Autodesk Fusion 360 part; units mm, degrees
(part 2 of 2)
  arc A35 (2.9933, 35.5014) -> (4.0928, 36.0294) centre (3.2566, 36.3621) ccw
  arc A36 (2.9933, 35.5014) -> (2.3013, 35.6868) centre (0, 25.7143) ccw
  arc A37 (1.6131, 36.6939) -> (2.3013, 35.6868) centre (2.5036, 36.5638) ccw
  line L18 (1.6131, 36.6939) -> (1.7553, 37.6675)
  spline S18 degree 5 poles (1.7553, 37.6675) (1.7565, 37.6761) (1.7588, 37.6933) (1.7613, 37.7191) (1.7631, 37.7537) (1.7633, 37.797) (1.7619, 37.8405) (1.7595, 37.8841) (1.7567, 37.9278) (1.7535, 37.9715) (1.7499, 38.0152) (1.7458, 38.059) (1.741, 38.1028) (1.7355, 38.1467) (1.7292, 38.1906) (1.7222, 38.2345) (1.7147, 38.2784) (1.7066, 38.3224) (1.698, 38.3663) (1.6891, 38.4103) (1.6797, 38.4543) (1.6698, 38.4982) (1.6595, 38.5422) (1.6487, 38.5862) (1.6374, 38.6301) (1.6257, 38.6741) (1.6135, 38.7181) (1.6009, 38.762) (1.5879, 38.8059) (1.5745, 38.8498) (1.5607, 38.8937) (1.5466, 38.9376) (1.532, 38.9814) (1.517, 39.0253) (1.5016, 39.0691) (1.4859, 39.1128) (1.4697, 39.1566) (1.4532, 39.2003) (1.4364, 39.244) (1.4192, 39.2876) (1.4016, 39.3312) (1.3836, 39.3748) (1.3654, 39.4183) (1.3467, 39.4618) (1.3277, 39.5053) (1.3084, 39.5487) (1.2887, 39.592) (1.2687, 39.6354) (1.2483, 39.6786) (1.2277, 39.7219) (1.2066, 39.765) (1.1853, 39.8081) (1.1636, 39.8512) (1.1416, 39.8942) (1.1193, 39.9372) (1.0967, 39.9801) (1.0738, 40.0229) (1.0505, 40.0657) (1.0269, 40.1084) (1.003, 40.151) (0.9788, 40.1936) (0.9543, 40.2361) (0.9295, 40.2786) (0.9044, 40.321) (0.879, 40.3633) (0.8533, 40.4055) (0.8273, 40.4477) (0.801, 40.4898) (0.7744, 40.5318) (0.7475, 40.5738) (0.7203, 40.6156) (0.6983, 40.6491) (0.6817, 40.6741) (0.6706, 40.6908) (0.665, 40.6991) knots 0 0 0 0 0 0 0.01428571 0.02857143 0.04285714 0.05714286 0.07142857 0.08571429 0.1 0.11428571 0.12857143 0.14285714 0.15714286 0.17142857 0.18571429 0.2 0.21428571 0.22857143 0.24285714 0.25714286 0.27142857 0.28571429 0.3 0.31428571 0.32857143 0.34285714 0.35714286 0.37142857 0.38571429 0.4 0.41428571 0.42857143 0.44285714 0.45714286 0.47142857 0.48571429 0.5 0.51428571 0.52857143 0.54285714 0.55714286 0.57142857 0.58571429 0.6 0.61428571 0.62857143 0.64285714 0.65714286 0.67142857 0.68571429 0.7 0.71428571 0.72857143 0.74285714 0.75714286 0.77142857 0.78571429 0.8 0.81428571 0.82857143 0.84285714 0.85714286 0.87142857 0.88571429 0.9 0.91428571 0.92857143 0.94285714 0.95714286 0.97142857 0.98571429 1 1 1 1 1 1
  arc A38 (0.665, 40.6991) -> (-0.665, 40.6991) centre (0, 25.7143) ccw
  spline S19 degree 5 poles (-0.665, 40.6991) (-0.6706, 40.6908) (-0.6817, 40.6741) (-0.6983, 40.6491) (-0.7203, 40.6156) (-0.7475, 40.5738) (-0.7744, 40.5318) (-0.801, 40.4898) (-0.8273, 40.4477) (-0.8533, 40.4055) (-0.879, 40.3633) (-0.9044, 40.321) (-0.9295, 40.2786) (-0.9543, 40.2361) (-0.9788, 40.1936) (-1.003, 40.151) (-1.0269, 40.1084) (-1.0505, 40.0657) (-1.0738, 40.0229) (-1.0967, 39.9801) (-1.1193, 39.9372) (-1.1416, 39.8942) (-1.1636, 39.8512) (-1.1853, 39.8081) (-1.2066, 39.765) (-1.2277, 39.7219) (-1.2483, 39.6786) (-1.2687, 39.6354) (-1.2887, 39.592) (-1.3084, 39.5487) (-1.3277, 39.5053) (-1.3467, 39.4618) (-1.3654, 39.4183) (-1.3836, 39.3748) (-1.4016, 39.3312) (-1.4192, 39.2876) (-1.4364, 39.244) (-1.4532, 39.2003) (-1.4697, 39.1566) (-1.4859, 39.1128) (-1.5016, 39.0691) (-1.517, 39.0253) (-1.532, 38.9814) (-1.5466, 38.9376) (-1.5607, 38.8937) (-1.5745, 38.8498) (-1.5879, 38.8059) (-1.6009, 38.762) (-1.6135, 38.7181) (-1.6257, 38.6741) (-1.6374, 38.6301) (-1.6487, 38.5862) (-1.6595, 38.5422) (-1.6698, 38.4982) (-1.6797, 38.4543) (-1.6891, 38.4103) (-1.698, 38.3663) (-1.7066, 38.3224) (-1.7147, 38.2784) (-1.7222, 38.2345) (-1.7292, 38.1906) (-1.7355, 38.1467) (-1.741, 38.1028) (-1.7458, 38.059) (-1.7499, 38.0152) (-1.7535, 37.9715) (-1.7567, 37.9278) (-1.7595, 37.8841) (-1.7619, 37.8405) (-1.7633, 37.797) (-1.7631, 37.7537) (-1.7613, 37.7191) (-1.7588, 37.6933) (-1.7565, 37.6761) (-1.7553, 37.6675) knots -1 -1 -1 -1 -1 -1 -0.98571429 -0.97142857 -0.95714286 -0.94285714 -0.92857143 -0.91428571 -0.9 -0.88571429 -0.87142857 -0.85714286 -0.84285714 -0.82857143 -0.81428571 -0.8 -0.78571429 -0.77142857 -0.75714286 -0.74285714 -0.72857143 -0.71428571 -0.7 -0.68571429 -0.67142857 -0.65714286 -0.64285714 -0.62857143 -0.61428571 -0.6 -0.58571429 -0.57142857 -0.55714286 -0.54285714 -0.52857143 -0.51428571 -0.5 -0.48571429 -0.47142857 -0.45714286 -0.44285714 -0.42857143 -0.41428571 -0.4 -0.38571429 -0.37142857 -0.35714286 -0.34285714 -0.32857143 -0.31428571 -0.3 -0.28571429 -0.27142857 -0.25714286 -0.24285714 -0.22857143 -0.21428571 -0.2 -0.18571429 -0.17142857 -0.15714286 -0.14285714 -0.12857143 -0.11428571 -0.1 -0.08571429 -0.07142857 -0.05714286 -0.04285714 -0.02857143 -0.01428571 0 0 0 0 0 0
  line L19 (-1.7553, 37.6675) -> (-1.6131, 36.6939)
  arc A39 (-2.3013, 35.6868) -> (-1.6131, 36.6939) centre (-2.5036, 36.5638) ccw
  arc A40 (-2.3013, 35.6868) -> (-2.9933, 35.5014) centre (0, 25.7143) ccw
  arc A41 (-4.0928, 36.0294) -> (-2.9933, 35.5014) centre (-3.2566, 36.3621) ccw
  line L20 (-4.0928, 36.0294) -> (-4.4565, 36.9437)
  spline S20 degree 5 poles (-4.4565, 36.9437) (-4.4597, 36.9518) (-4.4664, 36.9678) (-4.4771, 36.9914) (-4.4928, 37.0223) (-4.5143, 37.0599) (-4.5373, 37.0969) (-4.5611, 37.1335) (-4.5854, 37.1698) (-4.6101, 37.2061) (-4.635, 37.2422) (-4.6605, 37.278) (-4.6865, 37.3136) (-4.7132, 37.3488) (-4.7406, 37.3837) (-4.7686, 37.4182) (-4.7971, 37.4525) (-4.8261, 37.4865) (-4.8555, 37.5203) (-4.8852, 37.5539) (-4.9153, 37.5873) (-4.9459, 37.6204) (-4.9768, 37.6533) (-5.0081, 37.686) (-5.0399, 37.7185) (-5.072, 37.7507) (-5.1045, 37.7826) (-5.1374, 37.8144) (-5.1706, 37.8459) (-5.2042, 37.8773) (-5.2381, 37.9084) (-5.2723, 37.9393) (-5.3068, 37.97) (-5.3417, 38.0004) (-5.3769, 38.0307) (-5.4125, 38.0607) (-5.4483, 38.0905) (-5.4845, 38.1201) (-5.5209, 38.1495) (-5.5576, 38.1787) (-5.5947, 38.2077) (-5.632, 38.2365) (-5.6696, 38.265) (-5.7075, 38.2934) (-5.7457, 38.3215) (-5.7841, 38.3494) (-5.8228, 38.3771) (-5.8618, 38.4046) (-5.9011, 38.4319) (-5.9406, 38.459) (-5.9804, 38.4859) (-6.0204, 38.5126) (-6.0607, 38.539) (-6.1013, 38.5653) (-6.1421, 38.5913) (-6.1831, 38.6172) (-6.2244, 38.6428) (-6.2659, 38.6682) (-6.3077, 38.6934) (-6.3497, 38.7184) (-6.392, 38.7432) (-6.4344, 38.7677) (-6.4771, 38.7921) (-6.5201, 38.8163) (-6.5632, 38.8402) (-6.6066, 38.8639) (-6.6502, 38.8874) (-6.6941, 38.9107) (-6.7381, 38.9338) (-6.7824, 38.9567) (-6.8269, 38.9794) (-6.8626, 38.9974) (-6.8895, 39.0107) (-6.9075, 39.0196) (-6.9165, 39.0241) knots 0 0 0 0 0 0 0.01428571 0.02857143 0.04285714 0.05714286 0.07142857 0.08571429 0.1 0.11428571 0.12857143 0.14285714 0.15714286 0.17142857 0.18571429 0.2 0.21428571 0.22857143 0.24285714 0.25714286 0.27142857 0.28571429 0.3 0.31428571 0.32857143 0.34285714 0.35714286 0.37142857 0.38571429 0.4 0.41428571 0.42857143 0.44285714 0.45714286 0.47142857 0.48571429 0.5 0.51428571 0.52857143 0.54285714 0.55714286 0.57142857 0.58571429 0.6 0.61428571 0.62857143 0.64285714 0.65714286 0.67142857 0.68571429 0.7 0.71428571 0.72857143 0.74285714 0.75714286 0.77142857 0.78571429 0.8 0.81428571 0.82857143 0.84285714 0.85714286 0.87142857 0.88571429 0.9 0.91428571 0.92857143 0.94285714 0.95714286 0.97142857 0.98571429 1 1 1 1 1 1
  arc A42 (-6.9165, 39.0241) -> (-8.0683, 38.359) centre (0, 25.7143) ccw
  spline S21 degree 5 poles (-8.0683, 38.359) (-8.069, 38.349) (-8.0703, 38.329) (-8.0722, 38.299) (-8.0745, 38.2591) (-8.0771, 38.2092) (-8.0794, 38.1594) (-8.0814, 38.1098) (-8.0832, 38.0601) (-8.0846, 38.0106) (-8.0857, 37.9612) (-8.0866, 37.9118) (-8.0871, 37.8626) (-8.0874, 37.8134) (-8.0874, 37.7643) (-8.087, 37.7153) (-8.0864, 37.6665) (-8.0854, 37.6177) (-8.0842, 37.569) (-8.0827, 37.5204) (-8.0808, 37.472) (-8.0787, 37.4236) (-8.0762, 37.3754) (-8.0734, 37.3273) (-8.0704, 37.2793) (-8.067, 37.2314) (-8.0633, 37.1836) (-8.0593, 37.1359) (-8.0549, 37.0884) (-8.0503, 37.041) (-8.0453, 36.9938) (-8.0401, 36.9466) (-8.0345, 36.8997) (-8.0285, 36.8528) (-8.0223, 36.8061) (-8.0157, 36.7596) (-8.0088, 36.7131) (-8.0016, 36.6669) (-7.994, 36.6208) (-7.9861, 36.5748) (-7.9778, 36.529) (-7.9692, 36.4834) (-7.9603, 36.438) (-7.951, 36.3927) (-7.9414, 36.3476) (-7.9314, 36.3027) (-7.921, 36.258) (-7.9103, 36.2135) (-7.8992, 36.1691) (-7.8878, 36.125) (-7.876, 36.081) (-7.8638, 36.0373) (-7.8511, 35.9938) (-7.8381, 35.9506) (-7.8246, 35.9076) (-7.8108, 35.8648) (-7.7966, 35.8223) (-7.782, 35.7799) (-7.767, 35.7378) (-7.7516, 35.696) (-7.7357, 35.6545) (-7.7192, 35.6133) (-7.702, 35.5726) (-7.6842, 35.5323) (-7.6659, 35.4923) (-7.6472, 35.4526) (-7.6281, 35.4132) (-7.6087, 35.3739) (-7.589, 35.335) (-7.5684, 35.2966) (-7.5466, 35.2591) (-7.5277, 35.2301) (-7.5126, 35.209) (-7.5021, 35.1953) (-7.4967, 35.1885) knots -1 -1 -1 -1 -1 -1 -0.98571429 -0.97142857 -0.95714286 -0.94285714 -0.92857143 -0.91428571 -0.9 -0.88571429 -0.87142857 -0.85714286 -0.84285714 -0.82857143 -0.81428571 -0.8 -0.78571429 -0.77142857 -0.75714286 -0.74285714 -0.72857143 -0.71428571 -0.7 -0.68571429 -0.67142857 -0.65714286 -0.64285714 -0.62857143 -0.61428571 -0.6 -0.58571429 -0.57142857 -0.55714286 -0.54285714 -0.52857143 -0.51428571 -0.5 -0.48571429 -0.47142857 -0.45714286 -0.44285714 -0.42857143 -0.41428571 -0.4 -0.38571429 -0.37142857 -0.35714286 -0.34285714 -0.32857143 -0.31428571 -0.3 -0.28571429 -0.27142857 -0.25714286 -0.24285714 -0.22857143 -0.21428571 -0.2 -0.18571429 -0.17142857 -0.15714286 -0.14285714 -0.12857143 -0.11428571 -0.1 -0.08571429 -0.07142857 -0.05714286 -0.04285714 -0.02857143 -0.01428571 0 0 0 0 0 0
  line L21 (-7.4967, 35.1885) -> (-6.8868, 34.4163)
  arc A43 (-6.9792, 33.2001) -> (-6.8868, 34.4163) centre (-7.593, 33.8584) ccw
  arc A44 (-6.9792, 33.2001) -> (-7.4859, 32.6935) centre (0, 25.7143) ccw
  arc A45 (-8.7021, 32.601) -> (-7.4859, 32.6935) centre (-8.1441, 33.3073) ccw
  line L22 (-8.7021, 32.601) -> (-9.4742, 33.211)
  spline S22 degree 5 poles (-9.4742, 33.211) (-9.481, 33.2164) (-9.4947, 33.2269) (-9.5158, 33.242) (-9.5448, 33.2609) (-9.5823, 33.2827) (-9.6207, 33.3032) (-9.6596, 33.323) (-9.6989, 33.3424) (-9.7383, 33.3614) (-9.778, 33.3802) (-9.818, 33.3985) (-9.8583, 33.4163) (-9.899, 33.4335) (-9.9402, 33.45) (-9.9817, 33.4659) (-10.0235, 33.4813) (-10.0656, 33.4962) (-10.108, 33.5108) (-10.1505, 33.5251) (-10.1933, 33.5389) (-10.2363, 33.5524) (-10.2795, 33.5654) (-10.323, 33.5781) (-10.3667, 33.5903) (-10.4107, 33.6021) (-10.4548, 33.6135) (-10.4992, 33.6246) (-10.5437, 33.6353) (-10.5884, 33.6456) (-10.6334, 33.6556) (-10.6784, 33.6653) (-10.7237, 33.6746) (-10.7691, 33.6835) (-10.8148, 33.6921) (-10.8605, 33.7004) (-10.9065, 33.7083) (-10.9526, 33.7158) (-10.9989, 33.7231) (-11.0453, 33.73) (-11.0918, 33.7366) (-11.1385, 33.7428) (-11.1854, 33.7487) (-11.2324, 33.7543) (-11.2795, 33.7596) (-11.3267, 33.7646) (-11.3741, 33.7692) (-11.4217, 33.7735) (-11.4693, 33.7776) (-11.5171, 33.7813) (-11.565, 33.7846) (-11.613, 33.7877) (-11.6611, 33.7905) (-11.7093, 33.7929) (-11.7577, 33.7951) (-11.8062, 33.7969) (-11.8547, 33.7985) (-11.9034, 33.7997) (-11.9522, 33.8007) (-12.0011, 33.8013) (-12.05, 33.8016) (-12.0991, 33.8017) (-12.1483, 33.8014) (-12.1975, 33.8009) (-12.2469, 33.8) (-12.2963, 33.7989) (-12.3459, 33.7975) (-12.3955, 33.7957) (-12.4452, 33.7937) (-12.4949, 33.7914) (-12.5448, 33.7888) (-12.5847, 33.7865) (-12.6147, 33.7846) (-12.6347, 33.7833) (-12.6448, 33.7826) knots 0 0 0 0 0 0 0.01428571 0.02857143 0.04285714 0.05714286 0.07142857 0.08571429 0.1 0.11428571 0.12857143 0.14285714 0.15714286 0.17142857 0.18571429 0.2 0.21428571 0.22857143 0.24285714 0.25714286 0.27142857 0.28571429 0.3 0.31428571 0.32857143 0.34285714 0.35714286 0.37142857 0.38571429 0.4 0.41428571 0.42857143 0.44285714 0.45714286 0.47142857 0.48571429 0.5 0.51428571 0.52857143 0.54285714 0.55714286 0.57142857 0.58571429 0.6 0.61428571 0.62857143 0.64285714 0.65714286 0.67142857 0.68571429 0.7 0.71428571 0.72857143 0.74285714 0.75714286 0.77142857 0.78571429 0.8 0.81428571 0.82857143 0.84285714 0.85714286 0.87142857 0.88571429 0.9 0.91428571 0.92857143 0.94285714 0.95714286 0.97142857 0.98571429 1 1 1 1 1 1
  arc A46 (-12.6448, 33.7826) -> (-13.3098, 32.6308) centre (0, 25.7143) ccw
  spline S23 degree 5 poles (-13.3098, 32.6308) (-13.3053, 32.6218) (-13.2965, 32.6038) (-13.2831, 32.5769) (-13.2651, 32.5411) (-13.2424, 32.4967) (-13.2196, 32.4524) (-13.1965, 32.4084) (-13.1732, 32.3645) (-13.1496, 32.3209) (-13.1259, 32.2775) (-13.102, 32.2344) (-13.0778, 32.1914) (-13.0535, 32.1487) (-13.0289, 32.1062) (-13.0041, 32.064) (-12.9791, 32.022) (-12.9539, 31.9802) (-12.9285, 31.9387) (-12.9029, 31.8974) (-12.877, 31.8563) (-12.851, 31.8155) (-12.8247, 31.775) (-12.7983, 31.7347) (-12.7716, 31.6947) (-12.7447, 31.6549) (-12.7176, 31.6154) (-12.6904, 31.5761) (-12.6628, 31.5371) (-12.6351, 31.4984) (-12.6072, 31.4599) (-12.5791, 31.4218) (-12.5507, 31.3839) (-12.5222, 31.3463) (-12.4934, 31.309) (-12.4644, 31.2719) (-12.4352, 31.2352) (-12.4058, 31.1987) (-12.3762, 31.1626) (-12.3464, 31.1268) (-12.3164, 31.0912) (-12.2861, 31.056) (-12.2557, 31.0211) (-12.225, 30.9866) (-12.1941, 30.9524) (-12.163, 30.9185) (-12.1316, 30.8849) (-12.1001, 30.8517) (-12.0684, 30.8188) (-12.0364, 30.7863) (-12.0042, 30.7541) (-11.9717, 30.7224) (-11.9391, 30.6911) (-11.9061, 30.6601) (-11.873, 30.6296) (-11.8396, 30.5995) (-11.806, 30.5698) (-11.7722, 30.5404) (-11.7382, 30.5114) (-11.7039, 30.4829) (-11.6694, 30.4549) (-11.6345, 30.4275) (-11.5993, 30.4008) (-11.5637, 30.3748) (-11.5279, 30.3493) (-11.4918, 30.3244) (-11.4556, 30.2997) (-11.4192, 30.2754) (-11.3826, 30.2516) (-11.3456, 30.2286) (-11.308, 30.2071) (-11.2771, 30.1914) (-11.2535, 30.1806) (-11.2375, 30.174) (-11.2295, 30.1708) knots -1 -1 -1 -1 -1 -1 -0.98571429 -0.97142857 -0.95714286 -0.94285714 -0.92857143 -0.91428571 -0.9 -0.88571429 -0.87142857 -0.85714286 -0.84285714 -0.82857143 -0.81428571 -0.8 -0.78571429 -0.77142857 -0.75714286 -0.74285714 -0.72857143 -0.71428571 -0.7 -0.68571429 -0.67142857 -0.65714286 -0.64285714 -0.62857143 -0.61428571 -0.6 -0.58571429 -0.57142857 -0.55714286 -0.54285714 -0.52857143 -0.51428571 -0.5 -0.48571429 -0.47142857 -0.45714286 -0.44285714 -0.42857143 -0.41428571 -0.4 -0.38571429 -0.37142857 -0.35714286 -0.34285714 -0.32857143 -0.31428571 -0.3 -0.28571429 -0.27142857 -0.25714286 -0.24285714 -0.22857143 -0.21428571 -0.2 -0.18571429 -0.17142857 -0.15714286 -0.14285714 -0.12857143 -0.11428571 -0.1 -0.08571429 -0.07142857 -0.05714286 -0.04285714 -0.02857143 -0.01428571 0 0 0 0 0 0
  line L23 (-11.2295, 30.1708) -> (-10.3151, 29.8071)
  arc A47 (-9.7871, 28.7076) -> (-10.3151, 29.8071) centre (-10.6478, 28.9708) ccw
  circle A48 centre (0, 25.7143) radius 3
  arc A49 (-1.6131, 14.7347) -> (-2.3013, 15.7417) centre (-2.5036, 14.8648) ccw
  line L24 (-1.6131, 14.7347) -> (-1.7553, 13.761)
  spline S24 degree 5 poles (-1.7553, 13.761) (-1.7565, 13.7525) (-1.7588, 13.7353) (-1.7613, 13.7095) (-1.7631, 13.6749) (-1.7633, 13.6315) (-1.7619, 13.588) (-1.7595, 13.5444) (-1.7567, 13.5008) (-1.7535, 13.4571) (-1.7499, 13.4133) (-1.7458, 13.3696) (-1.741, 13.3257) (-1.7355, 13.2819) (-1.7292, 13.238) (-1.7222, 13.1941) (-1.7147, 13.1502) (-1.7066, 13.1062) (-1.698, 13.0622) (-1.6891, 13.0183) (-1.6797, 12.9743) (-1.6698, 12.9303) (-1.6595, 12.8864) (-1.6487, 12.8424) (-1.6374, 12.7984) (-1.6257, 12.7545) (-1.6135, 12.7105) (-1.6009, 12.6666) (-1.5879, 12.6227) (-1.5745, 12.5787) (-1.5607, 12.5349) (-1.5466, 12.491) (-1.532, 12.4471) (-1.517, 12.4033) (-1.5016, 12.3595) (-1.4859, 12.3157) (-1.4697, 12.272) (-1.4532, 12.2283) (-1.4364, 12.1846) (-1.4192, 12.141) (-1.4016, 12.0973) (-1.3836, 12.0538) (-1.3654, 12.0102) (-1.3467, 11.9667) (-1.3277, 11.9233) (-1.3084, 11.8799) (-1.2887, 11.8365) (-1.2687, 11.7932) (-1.2483, 11.7499) (-1.2277, 11.7067) (-1.2066, 11.6636) (-1.1853, 11.6204) (-1.1636, 11.5774) (-1.1416, 11.5344) (-1.1193, 11.4914) (-1.0967, 11.4485) (-1.0738, 11.4057) (-1.0505, 11.3629) (-1.0269, 11.3202) (-1.003, 11.2776) (-0.9788, 11.235) (-0.9543, 11.1924) (-0.9295, 11.15) (-0.9044, 11.1076) (-0.879, 11.0653) (-0.8533, 11.023) (-0.8273, 10.9809) (-0.801, 10.9388) (-0.7744, 10.8968) (-0.7475, 10.8548) (-0.7203, 10.8129) (-0.6983, 10.7795) (-0.6817, 10.7545) (-0.6706, 10.7378) (-0.665, 10.7294) knots 0 0 0 0 0 0 0.01428571 0.02857143 0.04285714 0.05714286 0.07142857 0.08571429 0.1 0.11428571 0.12857143 0.14285714 0.15714286 0.17142857 0.18571429 0.2 0.21428571 0.22857143 0.24285714 0.25714286 0.27142857 0.28571429 0.3 0.31428571 0.32857143 0.34285714 0.35714286 0.37142857 0.38571429 0.4 0.41428571 0.42857143 0.44285714 0.45714286 0.47142857 0.48571429 0.5 0.51428571 0.52857143 0.54285714 0.55714286 0.57142857 0.58571429 0.6 0.61428571 0.62857143 0.64285714 0.65714286 0.67142857 0.68571429 0.7 0.71428571 0.72857143 0.74285714 0.75714286 0.77142857 0.78571429 0.8 0.81428571 0.82857143 0.84285714 0.85714286 0.87142857 0.88571429 0.9 0.91428571 0.92857143 0.94285714 0.95714286 0.97142857 0.98571429 1 1 1 1 1 1
  arc A50 (-0.665, 10.7294) -> (0.665, 10.7294) centre (0, 25.7143) ccw
  spline S25 degree 5 poles (0.665, 10.7294) (0.6706, 10.7378) (0.6817, 10.7545) (0.6983, 10.7795) (0.7203, 10.8129) (0.7475, 10.8548) (0.7744, 10.8968) (0.801, 10.9388) (0.8273, 10.9809) (0.8533, 11.023) (0.879, 11.0653) (0.9044, 11.1076) (0.9295, 11.15) (0.9543, 11.1924) (0.9788, 11.235) (1.003, 11.2776) (1.0269, 11.3202) (1.0505, 11.3629) (1.0738, 11.4057) (1.0967, 11.4485) (1.1193, 11.4914) (1.1416, 11.5344) (1.1636, 11.5774) (1.1853, 11.6204) (1.2066, 11.6636) (1.2277, 11.7067) (1.2483, 11.7499) (1.2687, 11.7932) (1.2887, 11.8365) (1.3084, 11.8799) (1.3277, 11.9233) (1.3467, 11.9667) (1.3654, 12.0102) (1.3836, 12.0538) (1.4016, 12.0973) (1.4192, 12.141) (1.4364, 12.1846) (1.4532, 12.2283) (1.4697, 12.272) (1.4859, 12.3157) (1.5016, 12.3595) (1.517, 12.4033) (1.532, 12.4471) (1.5466, 12.491) (1.5607, 12.5349) (1.5745, 12.5787) (1.5879, 12.6227) (1.6009, 12.6666) (1.6135, 12.7105) (1.6257, 12.7545) (1.6374, 12.7984) (1.6487, 12.8424) (1.6595, 12.8864) (1.6698, 12.9303) (1.6797, 12.9743) (1.6891, 13.0183) (1.698, 13.0622) (1.7066, 13.1062) (1.7147, 13.1502) (1.7222, 13.1941) (1.7292, 13.238) (1.7355, 13.2819) (1.741, 13.3257) (1.7458, 13.3696) (1.7499, 13.4133) (1.7535, 13.4571) (1.7567, 13.5008) (1.7595, 13.5444) (1.7619, 13.588) (1.7633, 13.6315) (1.7631, 13.6749) (1.7613, 13.7095) (1.7588, 13.7353) (1.7565, 13.7525) (1.7553, 13.761) knots -1 -1 -1 -1 -1 -1 -0.98571429 -0.97142857 -0.95714286 -0.94285714 -0.92857143 -0.91428571 -0.9 -0.88571429 -0.87142857 -0.85714286 -0.84285714 -0.82857143 -0.81428571 -0.8 -0.78571429 -0.77142857 -0.75714286 -0.74285714 -0.72857143 -0.71428571 -0.7 -0.68571429 -0.67142857 -0.65714286 -0.64285714 -0.62857143 -0.61428571 -0.6 -0.58571429 -0.57142857 -0.55714286 -0.54285714 -0.52857143 -0.51428571 -0.5 -0.48571429 -0.47142857 -0.45714286 -0.44285714 -0.42857143 -0.41428571 -0.4 -0.38571429 -0.37142857 -0.35714286 -0.34285714 -0.32857143 -0.31428571 -0.3 -0.28571429 -0.27142857 -0.25714286 -0.24285714 -0.22857143 -0.21428571 -0.2 -0.18571429 -0.17142857 -0.15714286 -0.14285714 -0.12857143 -0.11428571 -0.1 -0.08571429 -0.07142857 -0.05714286 -0.04285714 -0.02857143 -0.01428571 0 0 0 0 0 0
  line L25 (1.7553, 13.761) -> (1.6131, 14.7347)
  arc A51 (2.3013, 15.7417) -> (1.6131, 14.7347) centre (2.5036, 14.8648) ccw
  line L26 (2.3013, 15.7417) -> (-2.3013, 15.7417)
  line L27 (2.3013, 15.7417) -> (-97.6987, 15.7417)
  line L28 (-97.6987, 15.7417) -> (-97.6987, 25.7417)
  line L29 (-97.6987, 25.7417) -> (2.3013, 25.7417)
  line L30 (2.3013, 25.7417) -> (2.3013, 15.7417)
  dimension "d18" = 100
  dimension "d19" = 10
  constraint coincident A15.start A16.start
  constraint coincident A12.end A13.end
  constraint horizontal L27
  constraint vertical L28
  constraint horizontal L29
  constraint vertical L30
  measures "d18" distance of A15.start L27.end
  measures "d19" distance of A15.start L29.end
component "Spur Gear (12 teeth)" placed x (1, 0, 0) y (0, 1, 0) z (0, 0, 1) at (0, 0, 0)
hidden bodies 1
